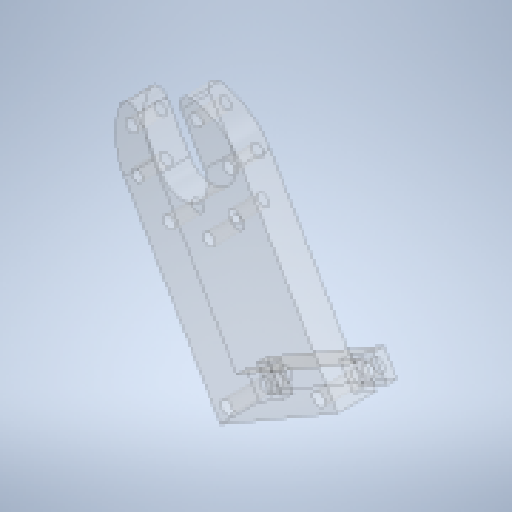
# Autodesk Inventor part: 부품47
Saved by Autodesk Inventor 2024 (Build 280153000, 153)
## iProperties
Created: 2024-09-07
Part Number: 부품47
Material: PMMA 플라스틱
Document SubType Name: Modeling
Designer: Eungang
Density: 1.188 g/cm^3
Appearance: 폴리카보네이트 - 선명
Mass: 7.60993 g
Surface Area: 35.839 cm^2
Volume: 6.40566 cm^3
Author: Eungang
Autodesk Inventor part; units mm, degrees
ref_plane "YZ Plane" through (0, 0, 0) normal (1, 0, 0) x (0, 1, 0)
ref_plane "XZ Plane" through (0, 0, 0) normal (0, 1, 0) x (-1, 0, 0)
ref_plane "XY Plane" through (0, 0, 0) normal (0, 0, 1) x (1, 0, 0)
sketch "스케치2" plane through (0, 0, 0) normal (0, 0, 1) x (1, 0, 0)
  circle A0 centre (0, 0) radius 14 projected
  arc A1 (-12.8234, 5.618) -> (-12.1163, -7.014) centre (0, 0) ccw projected
  line L0 (-12.1163, -7.014) -> (7.824, -41.4595) projected
  line L1 (7.824, -41.4595) -> (32.0565, -27.4315) projected
  line L2 (32.0565, -27.4315) -> (12.1163, 7.014) projected
  arc A2 (12.1163, 7.014) -> (1.5142, 13.9179) centre (0, 0) ccw projected
  circle A3 centre (9.5199, 5.511) radius 1.25 projected
  circle A4 centre (-9.5199, -5.511) radius 1.25 projected
  circle A5 centre (-10.6285, 2.8347) radius 1.25 projected
  circle A6 centre (28.2072, -26.7702) radius 1.35 projected
  circle A7 centre (9.1674, -37.7922) radius 1.35 projected
  circle A8 centre (2.8347, 10.6285) radius 1.25 projected
  circle A9 centre (-2.8347, -10.6285) radius 1.25 projected
  circle A10 centre (5.511, -9.5199) radius 1.25 projected
  circle A11 centre (10.6285, -2.8347) radius 1.25 projected
  circle A12 centre (0, 0) radius 7.25
  line L3 (-9.5199, -5.511) -> (9.5199, 5.511)
  line L4 (9.5199, 5.511) -> (-6.2745, -3.6323)
  arc A13 (-11.0126, 8.6443) -> (1.6585, 13.9014) centre (0, 0) ccw
  line L5 (3.9327, -21.2645) -> (16.4817, -14)
  circle A14 centre (9.5199, 5.511) radius 1.25
  circle A15 centre (-9.5199, -5.511) radius 1.25
  circle A16 centre (-10.6285, 2.8347) radius 1.25
  circle A17 centre (-5.511, 9.5199) radius 1.25
  circle A18 centre (2.8347, 10.6285) radius 1.25
  circle A19 centre (0, 0) radius 7.25
  line L6 (-16.4817, 14) -> (-3.9327, 21.2645)
  circle A20 centre (0, 0) radius 5.2
  line L7 (-4.5003, -2.6052) -> (-9.3099, 5.7031)
  line L8 (4.5003, 2.6052) -> (-0.3093, 10.9135)
  arc A21 (13.8078, -2.3119) -> (-2.0119, 13.8547) centre (0, 0) ccw
  arc A22 (-12.881, 5.4846) -> (-4.8714, -13.1251) centre (0, 0) ccw
  arc A23 (-9.3099, 5.7031) -> (-12.881, 5.4846) centre (-11.0408, 4.7011) ccw
  arc A24 (1.6585, 13.9014) -> (-0.3093, 10.9135) centre (1.4216, 11.9155) ccw
  line L9 (17.8441, -36.8125) -> (14.8381, -31.6198) projected
  line L10 (5.3181, -37.1308) -> (14.8381, -31.6198) projected
  line L11 (8.3241, -42.3235) -> (5.3181, -37.1308) projected
  line L12 (17.8441, -36.8125) -> (8.3241, -42.3235) projected
  circle A25 centre (9.1674, -37.7922) radius 1.35 projected
  line L13 (20.0307, -28.6138) -> (23.0367, -33.8065) projected
  line L14 (32.5567, -28.2955) -> (23.0367, -33.8065) projected
  line L15 (29.5507, -23.1028) -> (32.5567, -28.2955) projected
  line L16 (20.0307, -28.6138) -> (29.5507, -23.1028) projected
  circle A26 centre (28.2072, -26.7702) radius 1.35 projected
  line L17 (8.3606, -42.1868) -> (5.4548, -37.1673)
  line L18 (5.4548, -37.1673) -> (14.8016, -31.7564)
  line L19 (14.8016, -31.7564) -> (17.7074, -36.776)
  line L20 (17.7074, -36.776) -> (8.3606, -42.1868)
  line L21 (8.3606, -42.1868) -> (8.274, -42.2369)
  line L22 (8.274, -42.2369) -> (32.5066, -28.2089)
  point P0 (0, 0)
  point P1 (6.2745, 3.6323)
  point P2 (-0.2742, -13.9973)
  point P3 (12.2747, -6.7328)
  point P4 (0, 0)
  point P5 (0, 0)
  point P6 (-12.2747, 6.7328)
  point P7 (0.2742, 13.9973)
  point P8 (-12.881, 5.4846)
  point P9 (1.6585, 13.9014)
  dimension "d16" = 2
  dimension "d17" = 0.1
  constraints: 24 end point, 19 point on circle, 13 centre point, 9 point on line, 9 symmetric about line, 6 tangent, 2 coincident, 2 perpendicular, 1 equal radius, 9 other
  measures "d16" radius of A23
  measures "d17" distance between parallel lines of L12 L20
extrude "돌출1" add sketch "스케치2" along normal blind 6 contours A0 A23 L7 A12 L8 A24 | A0 L2 L16 L13 L1 L9 L10 L0 | L2 L1 L13 L16 | A12 L3 L8 | L10 L9 L1 L19 L18 L17 L0 | A12 L3 A20 | L7 L3 A12 | L1 L17 L18 L19 picked at (1.2989, -11.4658)
sketch "스케치8" plane through (0, 0, 0) normal (0, 0, -1) x (-1, 0, 0)
  circle A0 centre (9.5199, -5.511) radius 1.25 projected
  circle A1 centre (2.8347, -10.6285) radius 1.25 projected
  circle A2 centre (-5.511, -9.5199) radius 1.25 projected
  circle A3 centre (-10.6285, -2.8347) radius 1.25 projected
  circle A4 centre (-9.5199, 5.511) radius 1.25 projected
  circle A5 centre (-28.2072, -26.7702) radius 1.35 projected
  circle A6 centre (-9.1674, -37.7922) radius 1.35 projected
  line L0 (-7.824, -41.4595) -> (-32.0565, -27.4315) projected
  line L1 (12.1163, -7.014) -> (-7.824, -41.4595) projected
  arc A7 (12.1163, -7.014) -> (12.881, 5.4846) centre (0, 0) ccw projected
  arc A8 (12.881, 5.4846) -> (9.3099, 5.7031) centre (11.0408, 4.7011) ccw projected
  line L2 (4.5003, -2.6052) -> (9.3099, 5.7031) projected
  arc A9 (-4.5003, 2.6052) -> (4.5003, -2.6052) centre (0, 0) ccw projected
  line L3 (0.3093, 10.9135) -> (-4.5003, 2.6052) projected
  arc A10 (0.3093, 10.9135) -> (-1.6585, 13.9014) centre (-1.4216, 11.9155) ccw projected
  arc A11 (-1.6585, 13.9014) -> (-12.1163, 7.014) centre (0, 0) ccw projected
  line L4 (-32.0565, -27.4315) -> (-12.1163, 7.014) projected
  line L5 (-32.0565, -27.4315) -> (-7.824, -41.4595)
  line L6 (-34.4039, -32.4845) -> (-32.673, -33.4865) projected
  arc A12 (-32.673, -33.4865) -> (-29.5985, -32.6665) centre (-31.5458, -31.5392) ccw projected
  line L7 (-29.5985, -32.6665) -> (-28.5965, -30.9356) projected
  arc A13 (-27.2301, -30.5712) -> (-28.5965, -30.9356) centre (-27.7311, -31.4366) ccw projected
  line L8 (-27.2301, -30.5712) -> (-12.9502, -38.8377) projected
  arc A14 (-12.5858, -40.2041) -> (-12.9502, -38.8377) centre (-13.4512, -39.7031) ccw projected
  line L9 (-12.5858, -40.2041) -> (-13.5878, -41.935) projected
  arc A15 (-13.5878, -41.935) -> (-12.7678, -45.0095) centre (-11.6405, -43.0623) ccw projected
  line L10 (-12.7678, -45.0095) -> (-11.0369, -46.0115) projected
  arc A16 (-10.6724, -47.378) -> (-11.0369, -46.0115) centre (-11.5379, -46.877) ccw projected
  line L11 (-10.6724, -47.378) -> (-34.2195, -88.054) projected
  arc A17 (-35.5859, -88.4184) -> (-34.2195, -88.054) centre (-35.0849, -87.553) ccw projected
  line L12 (-35.5859, -88.4184) -> (-37.3168, -87.4164) projected
  arc A18 (-37.3168, -87.4164) -> (-40.3913, -88.2364) centre (-38.444, -89.3637) ccw projected
  line L13 (-40.3913, -88.2364) -> (-41.8943, -90.8328) projected
  line L14 (-36.918, -93.7135) -> (-41.8943, -90.8328) projected
  line L15 (-29.4982, -91.0759) -> (-36.918, -93.7135) projected
  line L16 (-2.8951, -45.1207) -> (-29.4982, -91.0759) projected
  line L17 (-4.3028, -37.3729) -> (-2.8951, -45.1207) projected
  line L18 (-30.2662, -22.3429) -> (-4.3028, -37.3729) projected
  line L19 (-37.686, -24.9805) -> (-30.2662, -22.3429) projected
  line L20 (-64.2892, -70.9357) -> (-37.686, -24.9805) projected
  line L21 (-62.8814, -78.6835) -> (-64.2892, -70.9357) projected
  line L22 (-57.9051, -81.5642) -> (-62.8814, -78.6835) projected
  line L23 (-57.9051, -81.5642) -> (-56.4021, -78.9679) projected
  arc A19 (-56.4021, -78.9679) -> (-57.2221, -75.8934) centre (-58.3493, -77.8406) ccw projected
  line L24 (-57.2221, -75.8934) -> (-58.953, -74.8914) projected
  arc A20 (-59.3174, -73.5249) -> (-58.953, -74.8914) centre (-58.452, -74.0259) ccw projected
  line L25 (-59.3174, -73.5249) -> (-35.7704, -32.8489) projected
  arc A21 (-34.4039, -32.4845) -> (-35.7704, -32.8489) centre (-34.9049, -33.3499) ccw projected
  circle A22 centre (-59.6114, -68.444) radius 1.35 projected
  circle A23 centre (-48.5894, -49.4042) radius 1.35 projected
  circle A24 centre (-28.2072, -26.7702) radius 1.35 projected
  circle A25 centre (-29.667, -85.7786) radius 1.35 projected
  circle A26 centre (-18.6449, -66.7388) radius 1.35 projected
  circle A27 centre (-9.1674, -37.7922) radius 1.35 projected
  circle A28 centre (-37.5674, -30.3643) radius 1.35 projected
  circle A29 centre (-7.6229, -47.699) radius 1.35 projected
  point P0 (0, 0)
  point P1 (-29.4008, -22.8439)
  point P2 (-17.2574, -35.9986)
  point P3 (-5.1683, -36.8719)
  constraints: 2 end point, 1 collinear
extrude "돌출4" add sketch "스케치8" along normal blind 8.8 contours L0 L4 L18 L1
sketch "스케치9" plane through (29.4008, -22.8439, 0) normal (-0.5010009, 0.8654468, 0) x (0.8654468, 0.5010009, 0)
  line L0 (-26.35, 8.8) -> (-23.65, 8.8) projected
  line L1 (-23.65, -6) -> (-26.35, -6) projected
  line L2 (-25, 8.8) -> (-25, -6)
  line L3 (-25, -2.5) -> (-25, 8.8)
  line L4 (-25, 8.8) -> (-25, -2.5)
  line L5 (-25, 3.15) -> (-27.6, 3.15)
  line L6 (-25, 3.15) -> (-22.4, 3.15)
  line L7 (-22.4, 3.15) -> (-22.4, 2.05)
  line L8 (-22.4, 3.15) -> (-22.4, 4.25)
  line L9 (-22.4, 4.25) -> (-27.6, 4.25)
  line L10 (-27.6, 4.25) -> (-27.6, 2.05)
  line L11 (-27.6, 2.05) -> (-22.4, 2.05)
  line L12 (-22.4, 2.05) -> (-22.4, 4.25)
  line L13 (-28, 0) -> (-28, 8.8) projected
  line L14 (-27.6, 4.25) -> (-28, 4.25)
  line L15 (-28, 4.25) -> (-28, 2.05)
  line L16 (-28, 2.05) -> (-27.6, 2.05)
  line L17 (-27.6, 2.05) -> (-27.6, 4.25)
  line L18 (0, 0) -> (-28, 0)
  line L19 (-26.35, -6) -> (-26.35, 8.8) projected
  line L20 (-14, 0) -> (-14, 8.8)
  line L21 (-28, 8.8) -> (0, 8.8) projected
  line L22 (-3, 3.15) -> (-0.4, 3.15)
  line L23 (-3, 3.15) -> (-5.6, 3.15)
  line L24 (-5.6, 3.15) -> (-5.6, 2.05)
  line L25 (-5.6, 3.15) -> (-5.6, 4.25)
  line L26 (-5.6, 4.25) -> (-0.4, 4.25)
  line L27 (-0.4, 4.25) -> (-0.4, 2.05)
  line L28 (-0.4, 2.05) -> (-5.6, 2.05)
  line L29 (-5.6, 2.05) -> (-5.6, 4.25)
  line L30 (-0.4, 4.25) -> (0, 4.25)
  line L31 (0, 4.25) -> (0, 2.05)
  line L32 (0, 2.05) -> (-0.4, 2.05)
  line L33 (-0.4, 2.05) -> (-0.4, 4.25)
  point P0 (-5.6, 2.05)
  point P1 (-0.4, 2.05)
  dimension "d20" = 2.6
  dimension "d21" = 2.6
  dimension "d22" = 1.1
  dimension "d23" = 1.1
  constraints: 58 end point, 11 symmetric about line, 5 perpendicular, 4 midpoint, 4 parallel, 3 horizontal, 2 point on line, 2 vertical, 1 collinear
  measures "d20" distance of L5.start L5.end
  measures "d21" distance of L5.start L6.end
  measures "d22" distance of L6.end L7.end
  measures "d23" distance of L6.end L8.end
extrude "돌출5" cut sketch "스케치9" against normal up to next contours L19 L5 L10 L9 | L9 L2 L5 L19 | L9 L8 L6 L2 | L10 L16 L13 L14 | L19 L11 L10 L5 | L5 L2 L11 L19 | L6 L7 L11 L2 | L23 L25 L26 L27 L22 | L22 L27 L28 L24 L23 | L27 L30 L31 L32
